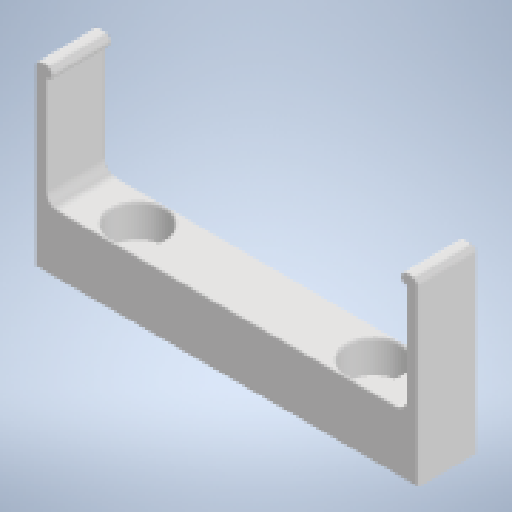
# Autodesk Inventor part: Top bot holder
Saved by Autodesk Inventor 2024 (Build 280153000, 153)
## iProperties
Created: 2024-04-04
Part Number: Top bot holder
Material: Generic
Document SubType Name: Modeling
Designer: jens1
Density: 1 g/cm^3
Appearance: Default
Author: jens1
Autodesk Inventor part; units mm, degrees
ref_plane "YZ Plane" through (0, 0, 0) normal (1, 0, 0) x (0, 1, 0)
ref_plane "XZ Plane" through (0, 0, 0) normal (0, 1, 0) x (-1, 0, 0)
ref_plane "XY Plane" through (0, 0, 0) normal (0, 0, 1) x (1, 0, 0)
sketch "Sketch1" plane through (0, 0, 0) normal (0, 0, 1) x (1, 0, 0)
  line L0 (0, 0) -> (65, 0)
  line L1 (65, 0) -> (65, 10)
  line L2 (65, 10) -> (0, 10)
  line L3 (0, 10) -> (0, 0)
  line L4 (0, 10) -> (2, 10)
  line L5 (2, 10) -> (2, 30.5)
  line L6 (2, 30.5) -> (0, 30.5)
  line L7 (0, 30.5) -> (0, 10)
  circle A0 centre (2, 29.5) radius 1
  line L8 (65, 10) -> (63, 10)
  line L9 (63, 10) -> (63, 30.5)
  line L10 (63, 30.5) -> (65, 30.5)
  line L11 (65, 30.5) -> (65, 10)
  circle A1 centre (63, 29.5) radius 1
  point P0 (63, 28.5)
  point P1 (2, 28.5)
  dimension "d4" = 2
  dimension "d7" = 2
  dimension "d0" = 65
  dimension "d1" = 10
  dimension "d2" = 2
  dimension "d3" = 20.5
  dimension "d5" = 2
  dimension "d6" = 20.5
  constraints: 24 end point, 6 parallel, 3 horizontal, 3 perpendicular, 2 point on line, 6 other
  measures "d0" distance of L2.end L1.end
  measures "d1" distance of L1.end L0.end
  measures "d2" distance of L6.end L5.end
  measures "d3" distance of L5.end L4.end
  measures "d5" distance of L9.end L10.end
  measures "d6" distance of L8.end L9.end
extrude "Extrusion1" add sketch "Sketch1" along normal blind 10
fillet "Fillet1" radius 2 2 edges at (2, 10, 5) (63, 10, 5)
fillet "Fillet2" radius 1 2 edges at (0, 30.5, 5) (65, 30.5, 5)
sketch "Sketch2" plane through (4, 10, 0) normal (0, 1, 0) x (1, 0, 0)
  line L0 (-4, 0) -> (61, 0) projected
  line L1 (61, 0) -> (61, -10) projected
  line L2 (-4, -10) -> (61, -10) projected
  line L3 (-4, 0) -> (-4, -10) projected
  point P0 (8.5, -5)
  point P1 (48.5, -5)
  dimension "d12" = 0
  dimension "d13" = 40
  dimension "d14" = 12.5
  dimension "d15" = 5
  measures "d12" vertical distance of point (48.5, -5) point (8.5, -5)
  measures "d13" distance of point (8.5, -5) point (48.5, -5)
  measures "d14" distance from line of L3 point (8.5, -5)
  measures "d15" distance from line of L0 point (48.5, -5)
hole "Hole1" at (12.5, 10, 5) at (52.5, 10, 5) direction (0, -1, 0) diameter 5.5 end through all counterbore diameter 9 counterbore depth 5.5
chamfer "Chamfer1" distance 0.25 angle 45 2 edges at (12.5, 10, 0.5) (52.5, 10, 0.5)
chamfer "Chamfer2" distance 0.25 angle 45 2 edges at (12.5, 4.5, 2.25) (52.5, 4.5, 2.25)
fillet "Fillet3" radius 0.25 14 edges at (0.2929, 30.2071, 10) (1.5, 30.5, 10) (3, 29.5, 10) (0, 14.75, 10) (2.5858, 10.5858, 10) (2, 20.25, 10) (62.4142, 10.5858, 10) (63, 20.25, 10) (32.5, 10, 10) (64.7071, 30.2071, 10) (63.5, 30.5, 10) (62, 29.5, 10) (65, 14.75, 10) (32.5, 0, 10)
fillet "Fillet4" radius 0.25 14 edges at (2.5858, 10.5858, 0) (2, 20.25, 0) (62.4142, 10.5858, 0) (63, 20.25, 0) (32.5, 10, 0) (64.7071, 30.2071, 0) (63.5, 30.5, 0) (62, 29.5, 0) (65, 14.75, 0) (32.5, 0, 0) (0.2929, 30.2071, 0) (1.5, 30.5, 0) (3, 29.5, 0) (0, 14.75, 0)
body "Solid1"
